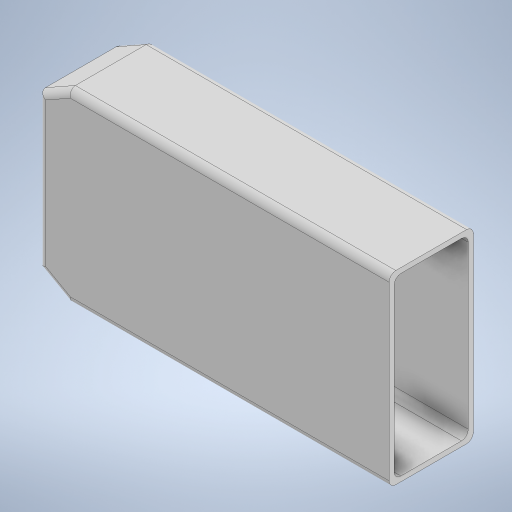
# Autodesk Inventor part: np2_headstage_box
Saved by Autodesk Inventor 2023.3 (Build 273359000, 359)
## iProperties
Created: 2023-11-21
Part Number: np2_headstage_box
Material: Generic
Document SubType Name: Modeling
Designer: mmelin
Density: 1 g/cm^3
Appearance: Default
Author: mmelin
Autodesk Inventor part; units mm, degrees
ref_plane "YZ Plane" through (0, 0, 0) normal (1, 0, 0) x (0, 1, 0)
ref_plane "XZ Plane" through (0, 0, 0) normal (0, 1, 0) x (-1, 0, 0)
ref_plane "XY Plane" through (0, 0, 0) normal (0, 0, 1) x (1, 0, 0)
sketch "Sketch1" plane through (0, 0, 0) normal (0, 0, 1) x (1, 0, 0)
  line L0 (0, -11) -> (-19, -11)
  line L1 (-19, -11) -> (-19, -10.7)
  line L2 (-19, -10.7) -> (0, -10.7)
  line L3 (0, -10.7) -> (0, -11)
  line L4 (0, -0.3) -> (-19, -0.3)
  line L5 (-19, -0.3) -> (-19, 0)
  line L6 (-19, 0) -> (0, 0)
  line L7 (0, 0) -> (0, -0.3)
  line L8 (-20.377, -10) -> (-20.777, -10)
  line L9 (-20.777, -10) -> (-20.777, -1)
  line L10 (-20.777, -1) -> (-20.377, -1)
  line L11 (-20.377, -1) -> (-20.377, -10)
  line L12 (-20.377, -10) -> (-19, -10.7)
  line L13 (-19, -11) -> (-20.777, -10)
  line L14 (-20.777, -1) -> (-19, 0)
  line L15 (-20.377, -1) -> (-19, -0.3)
  dimension "d0" = 0.3
  dimension "d1" = 19
  dimension "d2" = 10.4
  dimension "d3" = 0.4
  dimension "d4" = 1.777
  dimension "d5" = 0.7
  dimension "d6" = 0.7
  constraints: 32 end point, 6 parallel, 3 horizontal, 3 perpendicular, 2 collinear, 1 coincident, 1 point on line
  measures "d0" distance of L2.end L0.start
  measures "d1" distance of L1.end L2.end
  measures "d2" distance between parallel lines of L4 L2
  measures "d3" distance of L8.start L8.end
  measures "d4" distance between parallel lines of L9 L1
  measures "d5" distance between parallel lines of L8 L2
  measures "d6" distance between parallel lines of L4 L10
extrude "Extrusion1" add sketch "Sketch1" along normal blind 5
sketch "Sketch2" plane through (-19, -10.7, 0) normal (0, 1, 0) x (1, 0, 0)
  line L0 (3.5, -3.6) -> (3.1, -3.6)
  line L1 (3.1, -3.6) -> (3.1, -1.4)
  line L2 (3.1, -1.4) -> (3.5, -1.4)
  line L3 (3.5, -1.4) -> (3.5, -3.6)
  line L4 (3.5, -3.6) -> (3.5, -5) construction
  line L5 (19, -5) -> (0, -5) construction
  line L6 (3.5, -1.4) -> (3.5, 0) construction
  line L7 (19, 0) -> (0, 0) construction
  line L8 (19, 0) -> (19, -5) construction
  dimension "d9" = 0.4
  dimension "d10" = 1.4
  dimension "d11" = 15.5
  constraints: 12 end point, 3 point on line, 2 parallel, 1 collinear, 1 horizontal, 1 perpendicular, 1 vertical
  measures "d9" distance of L0.start L0.end
  measures "d10" distance of L2.end L6.end
  measures "d11" distance between parallel lines of L8 L3
extrude "Extrusion2" add sketch "Sketch2" along normal blind 0.5
sketch "Sketch3" plane through (-19, -0.3, 0) normal (0, -1, 0) x (1, 0, 0)
  line L0 (3.5, 1.4) -> (3.1, 1.4) projected
  line L1 (3.1, 1.4) -> (3.1, 3.6) projected
  line L2 (3.1, 3.6) -> (3.5, 3.6) projected
  line L3 (3.5, 3.6) -> (3.5, 1.4) projected
  point P0 (19, 0)
extrude "Extrusion3" add sketch "Sketch3" along normal blind 0.5
sketch "Sketch4" plane through (0, -0.3, 0) normal (1, 0, 0) x (0, 0, -1)
  line L0 (0, -10.4) -> (-5, -10.4) projected
  line L1 (0, 0) -> (-5, 0) projected
  line L2 (-5, -10.4) -> (-4.7, -10.4)
  line L3 (-4.7, -10.4) -> (-4.7, 0)
  line L4 (-4.7, 0) -> (-5, 0)
  line L5 (-5, 0) -> (-5, -10.4)
  line L6 (0, 0) -> (-0.3, 0)
  line L7 (-0.3, 0) -> (-0.3, -10.4)
  line L8 (-0.3, -10.4) -> (0, -10.4)
  line L9 (0, -10.4) -> (0, 0)
  point P0 (0, 0.3)
  point P1 (-0.3, 0)
  dimension "d16" = 0.3
  dimension "d17" = 0.3
  constraints: 16 end point, 4 parallel, 2 horizontal, 2 perpendicular, 2 point on line
  measures "d16" distance between parallel lines of L7 L9
  measures "d17" distance between parallel lines of L5 L3
extrude "Extrusion4" add sketch "Sketch4" against normal up to next contours L0 L7 L1 L9 | L0 L5 L1 L3
fillet "Fillet1" radius 0.4 18 edges at (-20.777, -5.5, 0) (-19.8885, -10.5, 0) (-19.8885, -10.5, 5) (-20.777, -5.5, 5) (-19.8885, -0.5, 0) (-19.8885, -0.5, 5) (-9.5, 0, 5) (-9.5, 0, 0) (-9.5, -11, 5) (-9.5, -11, 0) (-9.5, -10.7, 0.3) (-19, -10.7, 2.5) (-20.377, -10, 2.5) (-20.377, -1, 2.5) (-19, -0.3, 2.5) (-9.5, -0.3, 0.3) (-9.5, -0.3, 4.7) (-9.5, -10.7, 4.7)
equation "\"d17\" = d16"
body "Solid1"
